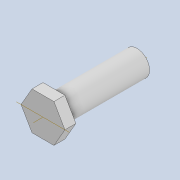
# Autodesk Inventor part: sruba m8
Saved by Autodesk Inventor 2021 (Build 250183000, 183)
## iProperties
Created: 2025-11-30
Part Number: sruba m8
Material: Generic
Document SubType Name: Modeling
Designer: huber
Density: 1 g/cm^3
Appearance: Default
Author: huber
Autodesk Inventor part; units mm, degrees
ref_plane "YZ Plane" through (0, 0, 0) normal (1, 0, 0) x (0, 1, 0)
ref_plane "XZ Plane" through (0, 0, 0) normal (0, 1, 0) x (-1, 0, 0)
ref_plane "XY Plane" through (0, 0, 0) normal (0, 0, 1) x (1, 0, 0)
sketch "Sketch1" plane through (0, 0, 0) normal (1, 0, 0) x (0, 1, 0)
  line L0 (0, 0) -> (7, 0)
  line L1 (7, 0) -> (7, -3.5)
  line L2 (7, -3.5) -> (4, -3.5)
  line L3 (4, -3.5) -> (4, -30)
  line L4 (4, -30) -> (0, -30)
  line L5 (0, -36) -> (0, 6) projected
  dimension "d0" = 3.5
  dimension "d1" = 4
  dimension "d2" = 30
  dimension "d3" = 7
  constraints: 10 end point, 4 perpendicular, 1 horizontal
  measures "d0" distance between parallel lines of L2 L0
  measures "d1" distance between parallel lines of L5 L3
  measures "d2" distance between parallel lines of L4 L0
  measures "d3" distance between parallel lines of L5 L1
revolve "Revolution1" add sketch "Sketch1" angle 360 about axis through (0, 0, -10) along (0, 0, 1)
sketch "Sketch2" plane through (0, 0, 0) normal (0, 0, 1) x (1, 0, 0)
  circle A0 centre (0, 0) radius 7 projected
  circle A1 centre (0, 0) radius 7 projected
  line L0 (7, 0) -> (3.5, -6.0622)
  line L1 (3.5, -6.0622) -> (-3.5, -6.0622)
  line L2 (-3.5, -6.0622) -> (-7, 0)
  line L3 (-7, 0) -> (-3.5, 6.0622)
  line L4 (-3.5, 6.0622) -> (3.5, 6.0622)
  line L5 (3.5, 6.0622) -> (7, 0)
  line L6 (-9.8, 0) -> (9.8, 0) projected
  point P0 (-7, 0)
  point P1 (-7, 0)
  constraints: 12 end point, 1 coincident, 1 horizontal alignment, 1 parallel, 14 other
extrude "Extrusion1" cut sketch "Sketch2" against normal blind 10 contours L5 A0 | A0 L0 | L4 A0 | A0 L1 | L2 A0 | A0 L3
body "Solid1"
